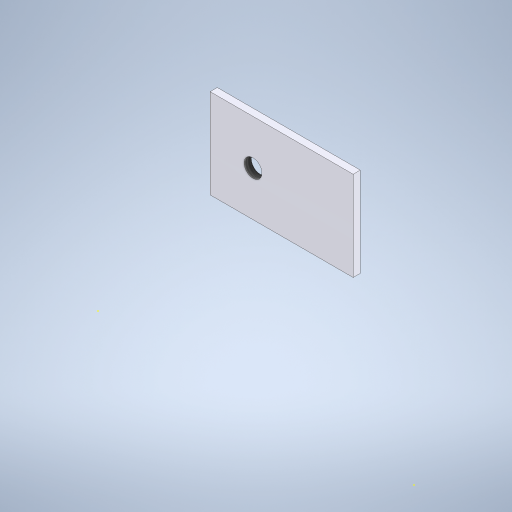
# Autodesk Inventor part: Peyangga Samping Kamera
Saved by Autodesk Inventor 2023 (Build 270158000, 158)
## iProperties
Created: 2025-05-22
Part Number: Peyangga Samping Kamera
Material: Generic
Document SubType Name: Modeling
Designer: ASUS
Density: 1 g/cm^3
Appearance: Default
Author: ASUS
Autodesk Inventor part; units mm, degrees
ref_plane "YZ Plane" through (0, 0, 0) normal (1, 0, 0) x (0, 1, 0)
ref_plane "XZ Plane" through (0, 0, 0) normal (0, 1, 0) x (-1, 0, 0)
ref_plane "XY Plane" through (0, 0, 0) normal (0, 0, 1) x (1, 0, 0)
sketch "Sketch1" plane through (0, 0, 0) normal (0, 0, 1) x (1, 0, 0)
  line L0 (31.3464, 73.7708) -> (86.3464, 73.7708)
  line L1 (86.3464, 73.7708) -> (86.3464, 38.7708)
  line L2 (86.3464, 38.7708) -> (31.3464, 38.7708)
  line L3 (31.3464, 38.7708) -> (31.3464, 73.7708)
  circle A0 centre (43.3464, 56.2708) radius 2.5
  point P0 (0, 0)
  dimension "d0" = 55
  dimension "d1" = 35
  dimension "d3" = 5
  constraints: 8 end point, 2 parallel, 1 centre point, 1 horizontal, 1 perpendicular
  measures "d0" distance of L1.end L2.end
  measures "d1" distance of L0.end L1.end
  measures "d3" diameter of A0
extrude "Extrusion1" add sketch "Sketch1" along normal blind 2
sketch "Sketch2" plane through (0, 0, 2) normal (0, 0, 1) x (1, 0, 0)
  point P0 (0, 0)
thread "Thread1" size "M5x0.8" class "6H" standard "ANSI Metric M Profile" length 43.6
sketch "Sketch3" plane through (86.3464, 38.7708, 0) normal (1, 0, 0) x (0, 0, -1)
  point P0 (0, -38.7708)
sketch "Sketch4" plane through (0, 0, 2) normal (0, 0, 1) x (1, 0, 0)
  point P0 (0, 0)
sketch "Sketch5" plane through (86.3464, 38.7708, 0) normal (1, 0, 0) x (0, 0, -1)
  line L0 (-2, 0) -> (-2, 35) projected
  line L1 (-2, 35) -> (0, 35)
  line L2 (0, 35) -> (0, 0)
  line L3 (0, 0) -> (-2, 0)
  line L4 (-2, 0) -> (-2, 35)
  point P0 (0, -38.7708)
  dimension "d8" = 2
  dimension "d9" = 35
  constraints: 8 end point, 2 parallel, 1 horizontal, 1 perpendicular
  measures "d8" distance of L2.end L3.end
  measures "d9" distance of L1.end L2.end
extrude "Extrusion2" cut sketch "Sketch5" against normal blind 15
sketch "Sketch6" plane through (0, 0, 2) normal (0, 0, 1) x (1, 0, 0)
  line L0 (31.3464, 38.7708) -> (71.3464, 38.7708) projected
  line L1 (31.3464, 38.7708) -> (71.3464, 38.7708)
  line L2 (71.3464, 38.7708) -> (71.3464, 43.7708)
  line L3 (71.3464, 43.7708) -> (31.3464, 43.7708)
  line L4 (31.3464, 43.7708) -> (31.3464, 38.7708)
  point P0 (0, 0)
  dimension "d12" = 40
  dimension "d13" = 5
  constraints: 8 end point, 2 parallel, 1 horizontal, 1 perpendicular
  measures "d12" distance of L3.end L2.end
  measures "d13" distance of L2.end L1.end
extrude "Extrusion3" cut sketch "Sketch6" against normal blind 15
sketch "Sketch7" plane through (0, 0, 0) normal (0, 0, -1) x (-1, 0, 0)
  line L0 (-71.3464, 73.7708) -> (-31.3464, 73.7708) projected
  line L1 (-71.3464, 73.7708) -> (-31.3464, 73.7708)
  line L2 (-31.3464, 73.7708) -> (-31.3464, 68.7708)
  line L3 (-31.3464, 68.7708) -> (-71.3464, 68.7708)
  line L4 (-71.3464, 68.7708) -> (-71.3464, 73.7708)
  point P0 (0, 0)
  dimension "d16" = 40
  dimension "d17" = 5
  constraints: 8 end point, 2 parallel, 1 horizontal, 1 perpendicular
  measures "d16" distance of L2.end L3.end
  measures "d17" distance of L1.end L2.end
extrude "Extrusion4" cut sketch "Sketch7" against normal blind 15
body "Solid1"
